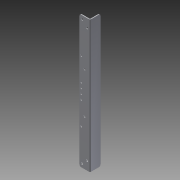
# Autodesk Inventor part: V5 Shooter Mounting Frame Channel Part 1
Saved by Autodesk Inventor 2014 SP1 (Build 180222100, 222)
## iProperties
Created: 2012-01-30
Part Number: V5 Shooter Mounting Frame Channel Part 1
Material: Aluminum-6061
Document SubType Name: Sheet Metal
Designer: Moses
Density: 2.71 g/cm^3
Sheet Metal Rule: Default
Mass: 329.664 g
Surface Area: 811.852 cm^2
Volume: 121.647 cm^3
Flat Pattern Width: 7.62 cm
Flat Pattern Length: 50.8 cm
Flat Pattern Area: 387.096 cm^2
Sheet Metal Width: 3.000 in
Sheet Metal Length: 20.000 in
Sheet Metal Area: 60.000 in^2
Appearance: Aluminum - Flat
Author: Moses
Autodesk Inventor part; units mm, degrees
ref_plane "YZ Plane" through (0, 0, 0) normal (1, 0, 0) x (0, 1, 0)
ref_plane "XZ Plane" through (0, 0, 0) normal (0, 1, 0) x (-1, 0, 0)
ref_plane "XY Plane" through (0, 0, 0) normal (0, 0, 1) x (1, 0, 0)
sketch "Sketch1" plane through (0, 0, 0) normal (0, 0, 1) x (1, 0, 0)
  line L0 (0, 0) -> (0, 508)
  line L1 (0, 508) -> (76.2, 508)
  line L2 (76.2, 508) -> (76.2, 0)
  line L3 (76.2, 0) -> (0, 0)
  line L4 (38.1, 508) -> (38.1, 0) construction
  line L5 (37.973, 12.7) -> (37.973, 6.35)
  line L6 (37.973, 6.35) -> (38.227, 6.35)
  line L7 (38.227, 6.35) -> (38.227, 12.7)
  line L8 (38.227, 12.7) -> (37.973, 12.7)
  line L9 (37.973, 29.5603) -> (37.973, 23.2103)
  line L10 (37.973, 23.2103) -> (38.227, 23.2103)
  line L11 (38.227, 23.2103) -> (38.227, 29.5603)
  line L12 (38.227, 29.5603) -> (37.973, 29.5603)
  line L13 (37.973, 46.4207) -> (37.973, 40.0707)
  line L14 (37.973, 40.0707) -> (38.227, 40.0707)
  line L15 (38.227, 40.0707) -> (38.227, 46.4207)
  line L16 (38.227, 46.4207) -> (37.973, 46.4207)
  line L17 (37.973, 63.281) -> (37.973, 56.931)
  line L18 (37.973, 56.931) -> (38.227, 56.931)
  line L19 (38.227, 56.931) -> (38.227, 63.281)
  line L20 (38.227, 63.281) -> (37.973, 63.281)
  line L21 (37.973, 80.1414) -> (37.973, 73.7914)
  line L22 (37.973, 73.7914) -> (38.227, 73.7914)
  line L23 (38.227, 73.7914) -> (38.227, 80.1414)
  line L24 (38.227, 80.1414) -> (37.973, 80.1414)
  line L25 (37.973, 97.0017) -> (37.973, 90.6517)
  line L26 (37.973, 90.6517) -> (38.227, 90.6517)
  line L27 (38.227, 90.6517) -> (38.227, 97.0017)
  line L28 (38.227, 97.0017) -> (37.973, 97.0017)
  line L29 (37.973, 113.8621) -> (37.973, 107.5121)
  line L30 (37.973, 107.5121) -> (38.227, 107.5121)
  line L31 (38.227, 107.5121) -> (38.227, 113.8621)
  line L32 (38.227, 113.8621) -> (37.973, 113.8621)
  line L33 (37.973, 130.7224) -> (37.973, 124.3724)
  line L34 (37.973, 124.3724) -> (38.227, 124.3724)
  line L35 (38.227, 124.3724) -> (38.227, 130.7224)
  line L36 (38.227, 130.7224) -> (37.973, 130.7224)
  line L37 (37.973, 147.5828) -> (37.973, 141.2328)
  line L38 (37.973, 141.2328) -> (38.227, 141.2328)
  line L39 (38.227, 141.2328) -> (38.227, 147.5828)
  line L40 (38.227, 147.5828) -> (37.973, 147.5828)
  line L41 (37.973, 164.4431) -> (37.973, 158.0931)
  line L42 (37.973, 158.0931) -> (38.227, 158.0931)
  line L43 (38.227, 158.0931) -> (38.227, 164.4431)
  line L44 (38.227, 164.4431) -> (37.973, 164.4431)
  line L45 (37.973, 181.3034) -> (37.973, 174.9534)
  line L46 (37.973, 174.9534) -> (38.227, 174.9534)
  line L47 (38.227, 174.9534) -> (38.227, 181.3034)
  line L48 (38.227, 181.3034) -> (37.973, 181.3034)
  line L49 (37.973, 198.1638) -> (37.973, 191.8138)
  line L50 (37.973, 191.8138) -> (38.227, 191.8138)
  line L51 (38.227, 191.8138) -> (38.227, 198.1638)
  line L52 (38.227, 198.1638) -> (37.973, 198.1638)
  line L53 (37.973, 215.0241) -> (37.973, 208.6741)
  line L54 (37.973, 208.6741) -> (38.227, 208.6741)
  line L55 (38.227, 208.6741) -> (38.227, 215.0241)
  line L56 (38.227, 215.0241) -> (37.973, 215.0241)
  line L57 (37.973, 231.8845) -> (37.973, 225.5345)
  line L58 (37.973, 225.5345) -> (38.227, 225.5345)
  line L59 (38.227, 225.5345) -> (38.227, 231.8845)
  line L60 (38.227, 231.8845) -> (37.973, 231.8845)
  line L61 (37.973, 248.7448) -> (37.973, 242.3948)
  line L62 (37.973, 242.3948) -> (38.227, 242.3948)
  line L63 (38.227, 242.3948) -> (38.227, 248.7448)
  line L64 (38.227, 248.7448) -> (37.973, 248.7448)
  line L65 (37.973, 265.6052) -> (37.973, 259.2552)
  line L66 (37.973, 259.2552) -> (38.227, 259.2552)
  line L67 (38.227, 259.2552) -> (38.227, 265.6052)
  line L68 (38.227, 265.6052) -> (37.973, 265.6052)
  line L69 (37.973, 282.4655) -> (37.973, 276.1155)
  line L70 (37.973, 276.1155) -> (38.227, 276.1155)
  line L71 (38.227, 276.1155) -> (38.227, 282.4655)
  line L72 (38.227, 282.4655) -> (37.973, 282.4655)
  line L73 (37.973, 299.3259) -> (37.973, 292.9759)
  line L74 (37.973, 292.9759) -> (38.227, 292.9759)
  line L75 (38.227, 292.9759) -> (38.227, 299.3259)
  line L76 (38.227, 299.3259) -> (37.973, 299.3259)
  line L77 (37.973, 316.1862) -> (37.973, 309.8362)
  line L78 (37.973, 309.8362) -> (38.227, 309.8362)
  line L79 (38.227, 309.8362) -> (38.227, 316.1862)
  line L80 (38.227, 316.1862) -> (37.973, 316.1862)
  line L81 (37.973, 333.0466) -> (37.973, 326.6966)
  line L82 (37.973, 326.6966) -> (38.227, 326.6966)
  line L83 (38.227, 326.6966) -> (38.227, 333.0466)
  line L84 (38.227, 333.0466) -> (37.973, 333.0466)
  line L85 (37.973, 349.9069) -> (37.973, 343.5569)
  line L86 (37.973, 343.5569) -> (38.227, 343.5569)
  line L87 (38.227, 343.5569) -> (38.227, 349.9069)
  line L88 (38.227, 349.9069) -> (37.973, 349.9069)
  line L89 (37.973, 366.7672) -> (37.973, 360.4172)
  line L90 (37.973, 360.4172) -> (38.227, 360.4172)
  line L91 (38.227, 360.4172) -> (38.227, 366.7672)
  line L92 (38.227, 366.7672) -> (37.973, 366.7672)
  line L93 (37.973, 383.6276) -> (37.973, 377.2776)
  line L94 (37.973, 377.2776) -> (38.227, 377.2776)
  line L95 (38.227, 377.2776) -> (38.227, 383.6276)
  line L96 (38.227, 383.6276) -> (37.973, 383.6276)
  line L97 (37.973, 400.4879) -> (37.973, 394.1379)
  line L98 (37.973, 394.1379) -> (38.227, 394.1379)
  line L99 (38.227, 394.1379) -> (38.227, 400.4879)
  line L100 (38.227, 400.4879) -> (37.973, 400.4879)
  line L101 (37.973, 417.3483) -> (37.973, 410.9983)
  line L102 (37.973, 410.9983) -> (38.227, 410.9983)
  line L103 (38.227, 410.9983) -> (38.227, 417.3483)
  line L104 (38.227, 417.3483) -> (37.973, 417.3483)
  line L105 (37.973, 434.2086) -> (37.973, 427.8586)
  line L106 (37.973, 427.8586) -> (38.227, 427.8586)
  line L107 (38.227, 427.8586) -> (38.227, 434.2086)
  line L108 (38.227, 434.2086) -> (37.973, 434.2086)
  line L109 (37.973, 451.069) -> (37.973, 444.719)
  line L110 (37.973, 444.719) -> (38.227, 444.719)
  line L111 (38.227, 444.719) -> (38.227, 451.069)
  line L112 (38.227, 451.069) -> (37.973, 451.069)
  line L113 (37.973, 467.9293) -> (37.973, 461.5793)
  line L114 (37.973, 461.5793) -> (38.227, 461.5793)
  line L115 (38.227, 461.5793) -> (38.227, 467.9293)
  line L116 (38.227, 467.9293) -> (37.973, 467.9293)
  line L117 (37.973, 484.7897) -> (37.973, 478.4397)
  line L118 (37.973, 478.4397) -> (38.227, 478.4397)
  line L119 (38.227, 478.4397) -> (38.227, 484.7897)
  line L120 (38.227, 484.7897) -> (37.973, 484.7897)
  line L121 (37.973, 501.65) -> (37.973, 495.3)
  line L122 (37.973, 495.3) -> (38.227, 495.3)
  line L123 (38.227, 495.3) -> (38.227, 501.65)
  line L124 (38.227, 501.65) -> (37.973, 501.65)
  line L125 (60.325, 508) -> (60.325, 3.175) construction
  circle A0 centre (60.325, 469.9) radius 11.1125
  circle A1 centre (60.325, 430.6455) radius 11.1125
  circle A2 centre (60.325, 391.3909) radius 11.1125
  circle A3 centre (60.325, 352.1364) radius 11.1125
  circle A4 centre (60.325, 312.8818) radius 11.1125
  circle A5 centre (60.325, 273.6273) radius 11.1125
  circle A6 centre (60.325, 234.3727) radius 11.1125
  circle A7 centre (60.325, 195.1182) radius 11.1125
  circle A8 centre (60.325, 155.8636) radius 11.1125
  circle A9 centre (60.325, 116.6091) radius 11.1125
  circle A10 centre (60.325, 77.3545) radius 11.1125
  circle A11 centre (60.325, 38.1) radius 11.1125
  point P0 (38.1, 6.35)
  point P1 (38.1, 23.2103)
  point P2 (38.1, 40.0707)
  point P3 (38.1, 56.931)
  point P4 (38.1, 73.7914)
  point P5 (38.1, 90.6517)
  point P6 (38.1, 107.5121)
  point P7 (38.1, 124.3724)
  point P8 (38.1, 141.2328)
  point P9 (38.1, 158.0931)
  point P10 (38.1, 174.9534)
  point P11 (38.1, 191.8138)
  point P12 (38.1, 208.6741)
  point P13 (38.1, 225.5345)
  point P14 (38.1, 242.3948)
  point P15 (38.1, 259.2552)
  point P16 (38.1, 276.1155)
  point P17 (38.1, 292.9759)
  point P18 (38.1, 309.8362)
  point P19 (38.1, 326.6966)
  point P20 (38.1, 343.5569)
  point P21 (38.1, 360.4172)
  point P22 (38.1, 377.2776)
  point P23 (38.1, 394.1379)
  point P24 (38.1, 410.9983)
  point P25 (38.1, 427.8586)
  point P26 (38.1, 444.719)
  point P27 (38.1, 461.5793)
  point P28 (38.1, 478.4397)
  point P29 (38.1, 495.3)
  dimension "d0" = 508
  dimension "d1" = 76.2
  dimension "d2" = 38.1
  dimension "d3" = 6.35
  dimension "d4" = 0.254
  dimension "d5" = 6.35
  dimension "d8" = 16.8603
  dimension "d47" = 22.225
  dimension "d48" = 22.225
  dimension "d49" = 38.1
  dimension "d52" = 39.2546
  constraints: 252 end point, 12 centre point, 6 perpendicular, 3 midpoint, 3 parallel, 3 point on line, 3 vertical, 283 other
  measures "d0" distance of L0.start L0.end
  measures "d1" distance of L0.end L1.end
  measures "d2" distance between parallel lines of L2 L4
  measures "d3" distance of L5.start L5.end
  measures "d4" distance of L5.end L6.end
  measures "d5" distance between parallel lines of L3 L6
  measures "d8" distance of L5.start L9.start
  measures "d47" distance between parallel lines of L125 L4
  measures "d48" diameter of A0
  measures "d49" distance from line of L1 A0.centre
  measures "d52" distance of A0.centre A1.centre
extrude "Plate1" add sketch "Sketch1" along normal blind 3.175 contours L0 L1 L2 L3 | L8 L7 L6 L5 | L12 L11 L10 L9 | L16 L15 L14 L13 | L20 L19 L18 L17 | L24 L23 L22 L21 | L28 L27 L26 L25 | L32 L31 L30 L29 | L36 L35 L34 L33 | L40 L39 L38 L37 | L44 L43 L42 L41 | L48 L47 L46 L45 | L52 L51 L50 L49 | L56 L55 L54 L53 | L60 L59 L58 L57 | L64 L63 L62 L61 | L68 L67 L66 L65 | L72 L71 L70 L69 | L76 L75 L74 L73 | L80 L79 L78 L77 | L84 L83 L82 L81 | L88 L87 L86 L85 | L92 L91 L90 L89 | L96 L95 L94 L93 | L100 L99 L98 L97 | L104 L103 L102 L101 | L108 L107 L106 L105 | L112 L111 L110 L109 | L116 L115 L114 L113 | L120 L119 L118 L117 | L124 L123 L122 L121 | A0 | A1 | A2 | A3 | A4 | A5 | A6 | A7 | A8 | A9 | A10 | A11
fold "Fold1" angle 90 bend radius 1.27 thickness 3.175 k factor 0.44 line from (38.1, 508, 0) to (38.1, 0, 0) line at bend centre moving side (1, 0, 0) folds toward (0, 0, -1)
sketch "Sketch2" plane through (0, 0, 3.175) normal (0, 0, 1) x (1, 0, 0)
  line L0 (36.0053, 0) -> (36.0053, 508) projected
  line L1 (0, 508) -> (36.0053, 508) projected
  line L2 (0, 0) -> (0, 508) projected
  line L3 (0, 254) -> (36.0053, 254) construction
  circle A0 centre (19.05, 332.75) radius 3.9751
  circle A1 centre (19.05, 175.25) radius 3.9751
  line L4 (40.4503, 508) -> (40.4503, 0) construction
  circle A2 centre (9.525, 494.03) radius 3.9751
  circle A3 centre (28.575, 474.98) radius 3.9751
  circle A4 centre (9.525, 13.97) radius 3.9751
  circle A5 centre (28.575, 33.02) radius 3.9751
  dimension "d20" = 7.9502
  dimension "d22" = 19.05
  dimension "d23" = 7.9502
  dimension "d24" = 7.9502
  dimension "d25" = 9.525
  dimension "d26" = 19.05
  dimension "d27" = 19.05
  dimension "d28" = 13.97
  dimension "d31" = 157.5
  constraints: 6 centre point, 3 symmetric about line, 2 end point, 2 midpoint, 3 other
  measures "d20" diameter of A0
  measures "d22" distance from line of L2 A0.centre
  measures "d23" diameter of A2
  measures "d24" diameter of A3
  measures "d25" distance from line of L2 A2.centre
  measures "d26" horizontal distance of A2.centre A3.centre
  measures "d27" horizontal distance of A2.centre A3.centre
  measures "d28" distance from line of L1 A2.centre
  measures "d31" distance of A0.centre A1.centre
extrude "Cut1" cut sketch "Sketch2" against normal blind 3.175
sketch "Sketch3" plane through (0, 0, 0) normal (0, 0, -1) x (-1, 0, 0)
  line L0 (-36.0053, 508) -> (-36.0053, 0) projected
  line L1 (0, 0) -> (0, 508) projected
  circle A0 centre (29.0293, 191.9287) radius 6.35 construction
  circle A1 centre (29.0293, 316.0712) radius 6.35 construction
  line L2 (29.0293, 191.9287) -> (-36.0053, 191.9287) construction
  line L3 (29.0293, 316.0712) -> (-36.0053, 316.0712) construction
  line L4 (0, 254) -> (-36.0053, 254) construction
  circle A2 centre (-6.35, 282.575) radius 3.3782
  circle A3 centre (-6.35, 263.525) radius 3.3782
  circle A4 centre (-6.35, 244.475) radius 3.3782
  circle A5 centre (-6.35, 225.425) radius 3.3782
  line L5 (-6.35, 263.525) -> (-6.35, 244.475) construction
  point P0 (-6.35, 254)
  dimension "d34" = 6.7564
  dimension "d38" = 19.05
  dimension "d43" = 6.35
  constraints: 8 end point, 4 centre point, 3 midpoint, 3 perpendicular, 3 point on line, 1 vertical, 6 other
  measures "d34" diameter of A2
  measures "d38" distance of A2.centre L5.start
  measures "d43" distance between parallel lines of L1 L5
extrude "Cut2" cut sketch "Sketch3" against normal blind 3.175
fillet "Corner Round1" radius 6.35 4 edges at (0, 508, 1.5875) (38.8628, 508, -37.2753) (0, 0, 1.5875) (38.8628, 0, -37.2753)
sketch "Sketch4" plane through (0, 0, 3.175) normal (0, 0, 1) x (1, 0, 0)
  line L0 (36.0053, 0) -> (36.0053, 508) projected
  line L1 (0, 6.35) -> (0, 501.65) projected
  circle A0 centre (6.35, 371.475) radius 3.3782
  circle A1 centre (6.35, 136.525) radius 3.3782
  line L2 (6.35, 136.525) -> (6.35, 371.475) construction
  line L3 (0, 254) -> (36.0053, 254) construction
  point P0 (0, 0)
  point P1 (6.35, 254)
  dimension "d57" = 6.7564
  dimension "d58" = 6.7564
  dimension "d59" = 6.35
  dimension "d60" = 234.95
  constraints: 4 end point, 3 midpoint, 2 centre point, 1 parallel, 1 point on line
  measures "d57" diameter of A0
  measures "d58" diameter of A1
  measures "d59" distance from line of L2.start L1
  measures "d60" distance of L2.start L2.end
extrude "Cut3" cut sketch "Sketch4" against normal blind 3.175
equation "\"d2\" = 0.5 * d1"
equation "\"d5\" = d3"
equation "\"d52\" = -0.181818 * d49 + 0.0909091 * d0"
equation "\"d14\" = BendReliefWidth"
equation "\"d15\" = BendReliefDepth"
equation "\"d16\" = MinimumRemnant"
equation "\"d17\" = BendRadius"
equation "\"d26\" = p1holespacing"
equation "\"d27\" = d26"
equation "\"d28\" = p1holedistedge"
equation "\"d29\" = Thickness"
equation "\"d34\" = d32"
equation "\"d44\" = Thickness"
equation "\"d61\" = Thickness"
equation "\"BendRadius\" = Thickness"
equation "\"BendReliefWidth\" = Thickness"
equation "\"BendReliefDepth\" = 0.5 * Thickness"
equation "\"CornerReliefSize\" = 4 * Thickness"
equation "\"MinimumRemnant\" = 2 * Thickness"
equation "\"TransitionRadius\" = BendRadius"
equation "\"JacobiRadiusSize\" = Thickness"
equation "\"GapSize\" = Thickness"
equation "\"d13\" = BendRadius"
equation "\"p1holespacing\" = 19.05"
equation "\"p1holedistedge\" = 13.97"
equation "\"Thickness\" = 3.175"
equation "\"d32\" = 6.7564"
body "Solid1"
